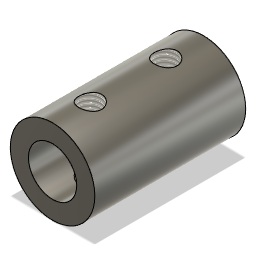
Coupler+Shaft (Autodesk Fusion 360 design; units mm, degrees)
Autodesk Fusion 360 part; units mm, degrees
note: some values were not read from the file. Set by a fixed rule: which face or edge a step refers to.
sketch "Sketch1" plane through (0, 0, 0) normal (0, 0, 1) x (1, 0, 0)
  circle A0 centre (0, 0) radius 2.5
  circle A1 centre (0, 0) radius 4
  circle A2 centre (0, 0) radius 7
  dimension "d1" = 5
  dimension "d2" = 8
  dimension "d3" = 14
  constraint coincident A0.centre A1.centre
  measures "d1" diameter of A0
  measures "d2" diameter of A1
  measures "d3" diameter of A2
extrude "Extrude1" add sketch "Sketch1" along normal blind 12.5 contours A2
extrude "Extrude2" add sketch "Sketch1" against normal blind 12.5 contours A1 | A2
sketch "Sketch2" plane through (0, 0, 0) normal (0, 1, 0) x (1, 0, 0)
  line L0 (7, 12.5) -> (-7, 12.5)
  line L1 (-7, -12.5) -> (7, -12.5)
  line L2 (0, 12.5) -> (0, 6.25)
  circle A0 centre (0, 6.25) radius 2.25
  line L3 (1.75, 0) -> (22.5, 0)
  circle A1 centre (0, -6.25) radius 2.25
  dimension "d8" = 6.25
  dimension "d9" = 4.5
  constraint midpoint L0 L2.start
  constraint perpendicular L0 L2
  constraint coincident L2.end A0.centre
  constraint symmetric A0 L3 A1
  measures "d8" distance of L2.start L2.end
  measures "d9" diameter of A0
extrude "Extrude3" cut sketch "Sketch2" along normal through all and the other way through all
thread "Thread1" "ISO Metric profile 4.5 M4.5x0.75 6H" major diameter 4.6131 minor diameter 3.7831 pitch 0.75 angle 60 resizes the face on face at (1.4853, 5.7997, 4.5599) on face at (0.8019, 5.4291, -8.3523) on face at (0.8297, -5.4199, -8.3414) on face at (1.4853, -5.7997, 4.5599)
